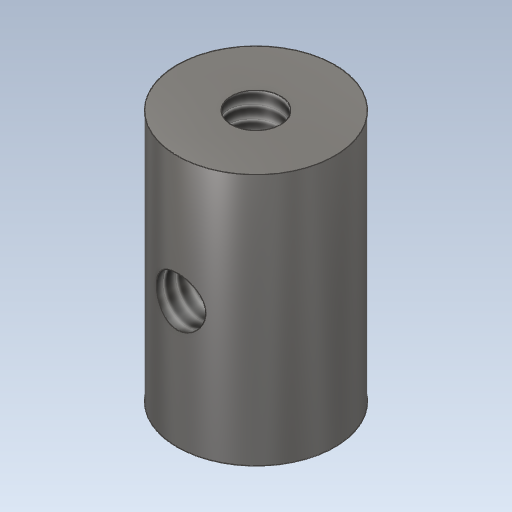
# Autodesk Inventor part: 200289
Saved by Autodesk Inventor 2020 (Build 240168000, 168)
## iProperties
Created: 2021-12-18
Part Number: 200289
Material: Steel, Carbon
Document SubType Name: Modeling
Designer: Byron Robotics
Mass: 33.8342 g
Surface Area: 21.242 cm^2
Volume: 4.31009 cm^3
Density: 7.85 g/cm^3
Appearance: Semi-Polished
Author: Byron Robotics
Autodesk Inventor part; units mm, degrees
ref_plane "YZ Plane" through (0, 0, 0) normal (1, 0, 0) x (0, 1, 0)
ref_plane "XZ Plane" through (0, 0, 0) normal (0, 1, 0) x (-1, 0, 0)
sketch "Sketch1" plane through (0, 0, 0) normal (0, 1, 0) x (-1, 0, 0)
  circle A0 centre (0, 0) radius 7.9375
  dimension "d0" = 15.875
  constraints: 1 centre point, 1 coincident
  measures "d0" diameter of A0
extrude "Extrusion1" add sketch "Sketch1" along normal blind 25.4
sketch "Sketch2" plane through (0, 25.4, 0) normal (0, 1, 0) x (1, 0, 0)
  point P0 (0, 0)
  point P1 (0, 0)
  constraints: 1 coincident
hole "Hole1" at (0, 25.4, 0) direction (0, -1, 0) diameter 4.9784 end through all thread size "1/4-20 UNC" class "2B" standard "ANSI Unified Screw Threads"
ref_plane "Work Plane1" through (0, 0, 7.9375) normal (0, 0, 1) x (1, 0, 0)
sketch "Sketch4" plane through (0, 0, 7.9375) normal (0, 0, 1) x (1, 0, 0)
  point P0 (0, 0)
  point P1 (0, 12.7)
  dimension "d11" = 12.7
  constraints: 1 vertical alignment
  measures "d11" distance of point (0, 0) point (0, 12.7)
hole "Hole2" at (0, 12.7, 7.9375) direction (0, 0, -1) diameter 4.9784 end through all thread size "1/4-20 UNC" class "2B" standard "ANSI Unified Screw Threads"
equation "\"d0\" = SlidingTensionerRoundDiameter"
equation "\"d1\" = ShapeWidth"
equation "\"d4\" = ShapeWidth"
equation "\"d11\" = 0.5 * ShapeWidth"
equation "\"d13\" = SlidingTensionerRoundDiameter"
equation "\"DrivebaseLength\" = 762"
equation "\"DrivebaseWidth\" = 660.4"
equation "\"ShapeHeight\" = 76.2"
equation "\"ShapeWidth\" = 25.4"
equation "\"ShapeThickness\" = 3.175"
equation "\"WheelDiameter\" = 152.4"
equation "\"WheelRadius\" = 76.2"
equation "\"WheelClearancetoFrame\" = 25.4"
equation "\"SlotLength\" = 88.9"
equation "\"SlotWidth\" = 15.9512"
equation "\"CenterAxleDrop\" = 3.175"
equation "\"CenterAxleXPosition\" = 381"
equation "\"CenterAxleYPosition\" = 25.4"
equation "\"Crossmember1Position\" = 203.2"
equation "\"Crossmember2Position\" = 203.2"
equation "\"CenterlineDrivebaseLength\" = 736.6"
equation "\"CenterlineDrivebaseWidth\" = 635"
equation "\"WheelDistanceFromEdge\" = 101.6"
equation "\"TensionAssemblyJointTravelLengthStart\" = -15.875"
equation "\"SlidingTensionerRoundClearance\" = 0.0762"
equation "\"CenterPointToTensionerRound\" = 28.575"
equation "\"SlidingTensionerRoundDiameter\" = 15.875"
equation "\"TensionAssemblyJointTravelLengthEnd\" = 15.875"
body "Solid1"
